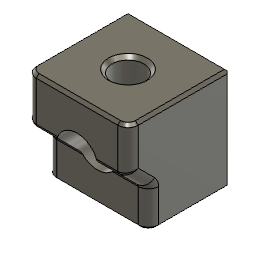
idler_end_kglm03_with_M3_gap_x2 v2 (Autodesk Fusion 360 design; units mm, degrees)
Autodesk Fusion 360 part; units mm, degrees
note: some values were not read from the file. Set by a fixed rule: which sketch regions a step uses.
sketch "Sketch1" plane through (0, 0, 0) normal (0, 0, 1) x (1, 0, 0)
  line L0 (7.5, 7.5) -> (-7.5, 7.5)
  line L1 (-7.5, 7.5) -> (-7.5, -7.5)
  line L2 (-7.5, -7.5) -> (7.5, -7.5)
  line L3 (7.5, -7.5) -> (7.5, 7.5)
  line L4 (7.5, 7.5) -> (-7.5, -7.5) construction
  line L5 (-7.5, 7.5) -> (7.5, -7.5) construction
  circle A0 centre (0, 0) radius 1.65
  circle A1 centre (0, 0) radius 3.1
  dimension "d1" = 15
  dimension "d2" = 15
  dimension "d3" = 3.3
  dimension "d9" = 6.2
  constraint horizontal L0
  constraint perpendicular L0 L1
  constraint parallel L0 L2
  constraint parallel L1 L3
  constraint coincident L4 A0.centre
  constraint coincident L5 A0.centre
  constraint coincident A0.centre A1.centre
  constraint concentric A0 A1
  measures "d1" distance of L0.start L2.end
  measures "d2" distance of L0.start L0.end
  measures "d3" diameter of A0
  measures "d9" diameter of A1
extrude "Extrude1" add sketch "Sketch1" along normal blind 15 contours L0 L1 L2 L3 | A1
sketch "Sketch2" plane through (0, 7.5, 0) normal (0, 1, 0) x (-1, 0, 0)
  line L0 (-7.5, 0) -> (7.5, 0)
  line L1 (7.5, 0) -> (7.5, 15)
  line L2 (7.5, 15) -> (-7.5, 15)
  line L3 (-7.5, 15) -> (-7.5, 0)
  circle A0 centre (0, 7.5) radius 2.35
  dimension "d6" = 4.7
  measures "d6" diameter of A0
extrude "Extrude2" cut sketch "Sketch2" against normal blind 4 contours A0
sketch "Sketch3" plane through (0, 0, 15) normal (0, 0, 1) x (1, 0, 0)
  circle A0 centre (0, 0) radius 1.65
  line L0 (7.5, -7.5) -> (7.5, 7.5)
  line L1 (7.5, 7.5) -> (-7.5, 7.5)
  line L2 (-7.5, 7.5) -> (-7.5, -7.5)
  line L3 (-7.5, -7.5) -> (7.5, -7.5)
  circle A1 centre (0, 0) radius 3.1
extrude "Extrude3" cut sketch "Sketch3" against normal blind 13 contours A1
sketch "Sketch4" plane through (-7.5, 0, 0) normal (-1, 0, 0) x (0, 0, 1)
  line L0 (0, 7.5) -> (0, -7.5)
  line L1 (0, -7.5) -> (15, -7.5)
  line L2 (15, -7.5) -> (15, 7.5)
  line L3 (15, 7.5) -> (0, 7.5)
  line L4 (15, 1) -> (12, -2)
  line L5 (0, -7.5) -> (12, -7.5)
  line L6 (15, 1) -> (15, 7.5)
  line L7 (5.15, 3.5) -> (9.85, 3.5)
  line L8 (5.15, 7.5) -> (9.85, 7.5)
  line L9 (12, -4) -> (0, -4)
  line L10 (12, -2) -> (12, -4)
  line L11 (12, -4) -> (12, -7.5)
  dimension "d12" = 12
  dimension "d20" = 3
  dimension "d21" = 3.5
  dimension "d22" = 135
  dimension "d23" = 5.5
  constraint coincident L2 L4.start
  constraint coincident L1 L5.end
  constraint coincident L0.end L1.start
  constraint coincident L2.end L3.start
  constraint coincident L0 L9.end
  constraint perpendicular L0 L9
  constraint vertical L10
  constraint vertical L11
  measures "d12" distance of L5.end L0.end
  measures "d20" distance of L2 L4.end
  measures "d21" distance of L5 L9
  measures "d22" angle of L4 L10
  measures "d23" distance of L5 L4.end
extrude "Extrude4" cut sketch "Sketch4" against normal blind 186 contours L1 L2 L4 L10 L11
fillet "Fillet1" radius 0.5 4 edges at (-5.2171, 1, 15) (5.2171, 1, 15) (4.9343, -2, 12) (-4.9343, -2, 12)
fillet "Fillet2" radius 1.5 10 edges at (7.5, 4.3536, 15) (7.5, 1.0158, 14.9619) (7.5, -0.5, 13.5) (7.5, -2.0158, 12.0381) (7.5, -4.8536, 12) (-7.5, 4.3536, 15) (-7.5, 1.0158, 14.9619) (-7.5, -0.5, 13.5) (-7.5, -2.0158, 12.0381) (-7.5, -4.8536, 12)
chamfer "Chamfer2" distance 0.5 angle 45 1 edges at (2.191, 7.5, 8.3498)
chamfer "Chamfer1" distance 0.4 angle 45 1 faces at (0.0411, -5.5485, 0)
chamfer "Chamfer3" distance 0.4 angle 45 1 faces at (2, -7.5, 4.2667)
sketch "Sketch5" plane through (0, -7.5, 0) normal (0, -1, 0) x (1, 0, 0)
  line L0 (7.1, 0.8) -> (7.1, 10.5)
  line L1 (-7.1, 10.5) -> (-7.1, 0.8)
  line L2 (-7.1, 0.8) -> (7.1, 0.8)
  circle A0 centre (0, 8) radius 2
  line L3 (-7.1, 0) -> (7.1, 0)
  arc A1 (7.1, 10.5) -> (6, 11.6) centre (6, 10.5) ccw
  line L4 (6, 11.6) -> (-6, 11.6)
  arc A2 (-6, 11.6) -> (-7.1, 10.5) centre (-6, 10.5) ccw
  line L5 (6, 12) -> (-6, 12)
  dimension "d28" = 8
  dimension "d29" = 4
  dimension "d34" = 4
  measures "d28" distance of A0.centre L3
  measures "d29" diameter of A0
  measures "d34" distance of A0.centre L5
extrude "Extrude5" cut sketch "Sketch5" against normal blind 2 contours A0
chamfer "Chamfer4" distance 0.4 angle 45 6 edges at (-1.8647, -7.5, 8.7232) (7.5, 7.5, 6.95) (7.0607, 7.5, 14.5607) (0, 7.5, 15) (-7.0607, 7.5, 14.5607) (-7.5, 7.5, 6.95)
sketch "Sketch6" plane through (0, 0, 0) normal (0, 0, -1) x (-1, 0, 0)
  circle A0 centre (0, 0) radius 2.05
  line L0 (-7.1, 7.1) -> (-7.1, -7.1)
  line L1 (-7.1, -7.1) -> (7.1, -7.1)
  line L2 (7.1, -7.1) -> (7.1, 7.1)
  line L3 (7.1, 7.1) -> (-7.1, 7.1)
  line L4 (-3.25, 6.7) -> (3.25, 6.7)
  line L5 (3.25, 6.7) -> (3.25, 3.7)
  line L6 (3.25, 3.7) -> (-3.25, 3.7)
  line L7 (-3.25, 3.7) -> (-3.25, 6.7)
  line L8 (-7.5, 7.1) -> (-7.5, -7.1)
  line L9 (7.1, 7.5) -> (-7.1, 7.5)
  dimension "d35" = 6.5
  dimension "d36" = 3
  dimension "d37" = 4.25
  dimension "d38" = 0.8
  constraint horizontal L4
  constraint vertical L5
  constraint horizontal L6
  constraint vertical L7
  measures "d35" distance of L4.start L4.end
  measures "d36" distance of L4.start L6.end
  measures "d37" distance of L7 L8
  measures "d38" distance of L4 L9
extrude "Extrude6" cut sketch "Sketch6" against normal blind 2 contours L4 L5 L6 L7
chamfer "Chamfer5" distance 0.25 angle 45 4 edges at (-3.25, 5.2, 0) (0, 6.7, 0) (0, 3.7, 0) (3.25, 5.2, 0)
equation "d10 = -15 mm + 2 mm"
named bodies: "idler_end_new_kglm03_x4"
